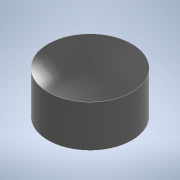
# Autodesk Inventor part: endcap
Saved by Autodesk Inventor 2021 (Build 250183000, 183)
## iProperties
Created: 2021-04-18
Part Number: endcap
Material: PVC, Unplasticized
Document SubType Name: Modeling
Designer: samlo
Density: 1.29 g/cm^3
Appearance: Dark Gray
Author: samlo
Autodesk Inventor part; units mm, degrees
ref_plane "YZ Plane" through (0, 0, 0) normal (1, 0, 0) x (0, 1, 0)
ref_plane "XZ Plane" through (0, 0, 0) normal (0, 1, 0) x (-1, 0, 0)
ref_plane "XY Plane" through (0, 0, 0) normal (0, 0, 1) x (1, 0, 0)
sketch "Sketch1" plane through (0, 0, 0) normal (0, 0, 1) x (1, 0, 0)
  line L0 (20, 0) -> (20, 21)
  line L1 (20, 21) -> (0, 21)
  line L2 (20, 0) -> (23, 0)
  line L3 (23, 0) -> (23, 23)
  line L4 (0, 21) -> (0, 25)
  arc A0 (23, 23) -> (0, 25) centre (-10.7095, -231.4093) ccw
  point P0 (0, 0)
  dimension "d0" = 20
  dimension "d1" = 23
  dimension "d2" = 0
  dimension "d3" = 21
  dimension "d5" = 25
  dimension "d7" = 23
  constraints: 10 end point, 2 perpendicular, 2 point on circle, 2 vertical, 1 centre point, 1 horizontal
  measures "d0" distance of L0.start point (0, 0)
  measures "d1" distance of L2.end point (0, 0)
  measures "d2" horizontal distance of L1.end point (0, 0)
  measures "d3" distance of L1.end point (0, 0)
  measures "d5" distance of point (0, 0) L4.end
  measures "d7" distance of L2.end L3.end
revolve "Revolution1" add sketch "Sketch1" angle 360 about axis through (0, 21, 0) along (0, 1, 0)
body "Solid1"
